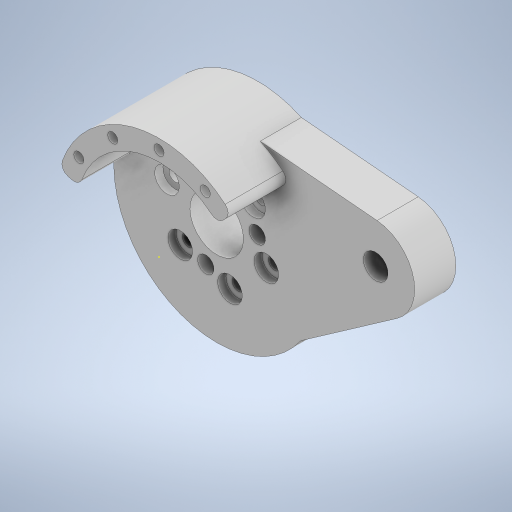
# Autodesk Inventor part: legparts_02(six)
Saved by Autodesk Inventor 2024.3 (Build 283343000, 343)
## iProperties
Created: 2024-10-20
Part Number: legparts_02(six)
Material: 一般
Document SubType Name: Modeling
Designer: 佐藤智貴
Density: 1 g/cm^3
Appearance: 既定
Mass: 23.5627 g
Surface Area: 98.5248 cm^2
Volume: 23.5627 cm^3
Author: 佐藤智貴
Autodesk Inventor part; units mm, degrees
ref_plane "YZ Plane" through (0, 0, 0) normal (1, 0, 0) x (0, 1, 0)
ref_plane "XZ Plane" through (0, 0, 0) normal (0, 1, 0) x (-1, 0, 0)
ref_plane "XY Plane" through (0, 0, 0) normal (0, 0, 1) x (1, 0, 0)
sketch "スケッチ1" plane through (0, 0, 0) normal (0, 0, 1) x (1, 0, 0)
  circle A0 centre (0, 0) radius 25
  circle A1 centre (0, 0) radius 20
  line L0 (0, 0) -> (-31.8868, 0)
  line L1 (0, 0) -> (-26.4988, 15.2991)
  line L2 (-26.4988, 15.2991) -> (0, 0)
  line L3 (0, 0) -> (27.9392, 16.1307)
  line L4 (0, 0) -> (0, 32.1911)
  point P0 (-25, 0)
  point P1 (-20, 0)
  point P2 (17.3205, 10)
  point P3 (21.6506, 12.5)
  dimension "d0" = 50
  dimension "d60" = 40
  dimension "d61" = 60
  dimension "d62" = 60
  constraints: 10 end point, 2 centre point, 2 coincident, 1 collinear, 1 horizontal, 1 vertical
  measures "d0" diameter of A0
  measures "d60" diameter of A1
  measures "d61" angle of L1 L4
  measures "d62" angle of L3 L4
extrude "押し出し1" add sketch "スケッチ1" along normal blind 14 contours L3 A1 L4 A0 | A0 L1 A1 L0 | L4 A1 L1 A0
sketch "スケッチ2" plane through (0, 0, 0) normal (0, 0, -1) x (0.9659258, 0.258819, 0)
  arc A0 (-24.1481, -6.4705) -> (24.1481, -6.4705) centre (0, 0) ccw projected
  line L0 (0, 25) -> (50, 6.8015)
  line L1 (0, -25) -> (50, -6.8015)
  line L2 (0, 0) -> (45.5986, 0)
  line L3 (0, 0) -> (0, 28.7036)
  line L4 (0, 0) -> (0, -28.8325)
  line L5 (50, -6.8015) -> (50, 6.8015)
  circle A1 centre (0, 0) radius 25
  circle A2 centre (40, 0) radius 3
  point P0 (16.0697, -19.1511)
  point P1 (12.8558, 15.3209)
  point P2 (0, -25)
  point P3 (-24.1481, -6.4705)
  point P4 (0, -25)
  point P5 (16.0697, 19.1511)
  dimension "d7" = 70
  dimension "d8" = 70
  dimension "d9" = 50
  dimension "d10" = 0
  dimension "d11" = 0
  dimension "d85" = 40
  dimension "d86" = 6
  dimension "d87" = 50
  constraints: 12 end point, 2 centre point, 2 point on circle, 2 vertical, 1 coincident, 1 concentric, 1 horizontal, 1 perpendicular, 1 point on line
  measures "d7" angle of L3 L0
  measures "d8" angle of L4 L1
  measures "d9" distance between parallel lines of L4 L5
  measures "d10" distance from line of L4 L1.start
  measures "d11" distance from line of L3 L0.start
  measures "d85" distance of point (0, 0) A2.centre
  measures "d86" diameter of A2
  measures "d87" diameter of A1
extrude "押し出し2" add sketch "スケッチ2" along normal blind 10
sketch "スケッチ3" plane through (0, 0, 14) normal (0, 0, 1) x (-0.9659258, -0.258819, 0)
  circle A0 centre (0, 0) radius 16.5
  circle A1 centre (0, 0) radius 12.5
  circle A2 centre (0, 0) radius 10.2
  line L0 (0, 0) -> (-30.0431, 0)
  line L1 (0, 0) -> (-11.9468, -6.8975)
  point P0 (-10.8253, -6.25)
  point P1 (0, -12.5)
  point P2 (10.8253, -6.25)
  point P3 (10.8253, 6.25)
  point P4 (0, 12.5)
  point P5 (-10.8253, 6.25)
  dimension "d16" = 25
  dimension "d15" = 33
  dimension "d17" = 20.4
  dimension "d19" = 30
  dimension "d22" = 360
  constraints: 4 end point, 2 centre point, 1 coincident, 1 horizontal, 1 point on line, 10 other
  measures "d15" diameter of A0
  measures "d17" diameter of A2
  measures "d19" angle of L0 L1
hole "穴1" at (8.8388, 8.8388, 14) at (-3.2352, 12.0741, 14) at (-12.0741, 3.2352, 14) at (-8.8388, -8.8388, 14) at (3.2352, -12.0741, 14) at (12.0741, -3.2352, 14) direction (0, 0, -1) diameter 3 end through all
sketch "スケッチ4" plane through (0, 0, 14) normal (0, 0, 1) x (-0.9659258, -0.258819, 0)
  circle A0 centre (0, 0) radius 10.2
  point P0 (-10.2, 0)
  point P1 (5.1, -8.8335)
  point P2 (5.1, 8.8335)
  dimension "d31" = 20.4
  dimension "d34" = 360
  constraints: 1 coincident, 1 horizontal alignment, 6 other
hole "穴2" at (9.8524, 2.64, 14) at (-7.2125, 7.2125, 14) at (-2.64, -9.8524, 14) direction (0, 0, -1) diameter 4 end through all
sketch "スケッチ6" plane through (0, 0, 14) normal (0, 0, 1) x (-0.9659258, -0.258819, 0)
  point P0 (0, 0)
sketch "スケッチ7" plane through (0, 0, -10) normal (0, 0, -1) x (0.9659258, 0.258819, 0)
  circle A0 centre (0, 0) radius 6.5
  dimension "d55" = 13
  constraints: 1 centre point, 1 coincident
  measures "d55" diameter of A0
extrude "押し出し3" cut sketch "スケッチ7" against normal through all
sketch "スケッチ9" plane through (0, 0, 14) normal (0, 0, 1) x (1, 0, 0)
  circle A0 centre (0, 0) radius 25
  circle A1 centre (0, 0) radius 20
  circle A2 centre (0, 0) radius 22.5
  line L0 (0, 0) -> (-21.7003, 0)
  line L1 (-19.4856, 11.25) -> (0, 0)
  line L2 (-11.25, 19.4856) -> (0, 0)
  line L3 (0, 22.5) -> (0, 0)
  line L4 (0, 0) -> (11.6379, 20.1574)
  line L5 (17.3205, 10) -> (21.6506, 12.5) projected
  point P0 (11.25, 19.4856)
  dimension "d64" = 50
  dimension "d65" = 40
  dimension "d63" = 45
  dimension "d66" = 30
  dimension "d67" = 60
  dimension "d68" = 90
  dimension "d69" = 30
  dimension "d88" = 150
  constraints: 10 end point, 4 point on circle, 3 coincident, 1 centre point, 1 horizontal, 1 point on line, 4 other
  measures "d63" diameter of A2
  measures "d66" angle of L0 L1
  measures "d67" angle of L0 L2
  measures "d68" angle of L0 L3
  measures "d69" angle of L3 L4
  measures "d88" angle of L0 L5
hole "穴4" at (0, 22.5, 14) at (-11.25, 19.4856, 14) at (-19.4856, 11.25, 14) at (11.25, 19.4856, 14) direction (0, 0, -1) diameter 2.459 end through all
sketch "スケッチ10" plane through (0, 0, 0) normal (0, 0, 1) x (0.9659258, 0.258819, 0)
  circle A0 centre (10.8253, 6.25) radius 1.5 projected
  circle A1 centre (10.8253, 6.25) radius 3
  circle A2 centre (0, 0) radius 12.5
  circle A3 centre (0, 12.5) radius 3
  circle A4 centre (-10.8253, 6.25) radius 3
  circle A5 centre (-10.8253, -6.25) radius 3
  circle A6 centre (0, -12.5) radius 3
  circle A7 centre (10.8253, -6.25) radius 3
  dimension "d78" = 6
  dimension "d81" = 360
  constraints: 6 centre point, 2 coincident, 16 other
  measures "d78" diameter of A1
extrude "押し出し5" cut sketch "スケッチ10" against normal blind 2 contours A0 A2 A1 | A0 A2 A1 | A3 A2 | A2 A3 | A7 A2 | A2 A7 | A4 A2 | A2 A4 | A6 A2 | A2 A6 | A5 A2 | A2 A5
sketch "スケッチ11" plane through (0, 0, 14) normal (0, 0, 1) x (1, 0, 0)
  circle A0 centre (38.637, 10.3528) radius 3 projected
  line L0 (0, 0) -> (38.637, 10.3528)
  line L1 (38.637, 10.3528) -> (-19.2634, -5.1616)
  circle A1 centre (0, 0) radius 25
  circle A2 centre (0, 0) radius 15
  line L2 (0, 0) -> (24.2052, 24.2052)
  line L3 (24.2052, 24.2052) -> (0, 0)
  line L4 (0, 0) -> (-32.0338, 8.5834)
  line L5 (0, 0) -> (-33.1646, 0)
  line L6 (0, 0) -> (25.9754, 14.9969)
  point P0 (-25, 0)
  point P1 (-15, 0)
  point P2 (-14.4889, 3.8823)
  point P3 (-24.1481, 6.4705)
  point P4 (12.9904, 7.5)
  point P5 (21.6506, 12.5)
  point P6 (17.6777, 17.6777)
  point P7 (10.6066, 10.6066)
  dimension "d90" = 50
  dimension "d91" = 30
  dimension "d92" = 30
  dimension "d93" = 30
  dimension "d94" = 15
  constraints: 14 end point, 2 centre point, 2 coincident, 1 collinear, 1 horizontal, 1 point on line
  measures "d90" diameter of A1
  measures "d91" diameter of A2
  measures "d92" angle of L0 L2
  measures "d93" angle of L1 L4
  measures "d94" angle of L0 L6
extrude "押し出し6" cut sketch "スケッチ11" against normal blind 14 contours L2 A1 L6 A2 | A2 L5 A1 L4
fillet "フィレット3" radius 2 5 edges at (-24.1481, 6.4705, 7) (-19.3185, 5.1764, 7) (17.6777, 17.6777, 7) (14.1421, 14.1421, 7) (-5.1764, 19.3185, 0)
fillet "フィレット4" radius 10 2 edges at (46.5359, 19.5107, -5) (50.0566, 6.3712, -5)
equation "\"d62\" = d61"
equation "\"d8\" = d7"
equation "\"d69\" = d66"
